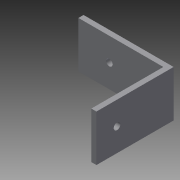
# Autodesk Inventor part: 000102 (revised)
Saved by Autodesk Inventor 2015 (Build 190159000, 159)
## iProperties
Created: 2015-05-11
Part Number: 000102 (revised)
Material: Generic
Document SubType Name: Modeling
Designer: Caitlynn
Density: 1 g/cm^3
Appearance: Default
Author: Caitlynn
Autodesk Inventor part; units mm, degrees
ref_plane "YZ Plane" through (0, 0, 0) normal (1, 0, 0) x (0, 1, 0)
ref_plane "XZ Plane" through (0, 0, 0) normal (0, 1, 0) x (-1, 0, 0)
ref_plane "XY Plane" through (0, 0, 0) normal (0, 0, 1) x (1, 0, 0)
sketch "Sketch1" plane through (0, 0, 0) normal (0, 0, 1) x (1, 0, 0)
  line L0 (0, 0) -> (44.45, 0)
  line L1 (44.45, 0) -> (44.45, 22.86)
  line L2 (44.45, 22.86) -> (0, 22.86)
  line L3 (0, 22.86) -> (0, 0)
  dimension "d0" = 22.86
  dimension "d1" = 44.45
  constraints: 8 end point, 2 parallel, 1 horizontal, 1 perpendicular
  measures "d0" distance of L2.end L0.start
  measures "d1" distance of L1.end L2.end
extrude "Extrusion1" add sketch "Sketch1" along normal blind 2.54
sketch "Sketch2" plane through (0, 0, 2.54) normal (0, 0, 1) x (1, 0, 0)
  line L0 (0, 0) -> (44.45, 0) projected
  line L1 (44.45, 22.86) -> (41.91, 22.86)
  line L2 (41.91, 22.86) -> (41.91, 0)
  line L3 (41.91, 0) -> (44.45, 0)
  line L4 (44.45, 0) -> (44.45, 22.86)
  dimension "d4" = 2.54
  constraints: 8 end point, 2 parallel, 1 horizontal, 1 perpendicular, 1 point on line
  measures "d4" distance of L3.end L2.end
extrude "Extrusion2" add sketch "Sketch2" along normal blind 35.56
sketch "Sketch4" plane through (0, 0, 2.54) normal (0, 0, 1) x (1, 0, 0)
  line L0 (-11.3987, 11.43) -> (43.7828, 11.43) construction
  line L1 (0, 0) -> (41.91, 0) construction
  line L2 (41.91, 0) -> (41.91, 22.86) construction
  line L3 (41.91, 22.86) -> (0, 22.86) construction
  line L4 (0, 22.86) -> (0, 0) construction
  line L5 (0, 0) -> (41.91, 0) construction
  point P0 (15.24, 11.43)
  dimension "d16" = 11.43
  dimension "d17" = 26.67
  constraints: 2 end point, 1 horizontal, 1 point on line
  measures "d16" distance between parallel lines of L1 L0
  measures "d17" distance from line of point (15.24, 11.43) L2
hole "Hole2" at (15.24, 11.43, 2.54) direction (0, 0, -1) diameter 3.2512 end through all
sketch "Sketch5" plane through (41.91, 0, 2.54) normal (-1, 0, 0) x (0, 0, 1)
  line L0 (24.13, 11.4617) -> (25.4, 11.4617)
  circle A0 centre (25.4, 11.4617) radius 1.6412
  line L1 (0, 0) -> (0, 22.86) projected
  point P0 (-2.54, 0)
  dimension "d25" = 1.27
  dimension "d28" = 25.4
  constraints: 2 end point, 1 centre point, 1 coincident, 1 horizontal
  measures "d25" distance of L0.start L0.end
  measures "d28" distance from line of L1 L0.end
extrude "Extrusion3" cut sketch "Sketch5" against normal blind 25.4
body "Solid1"
